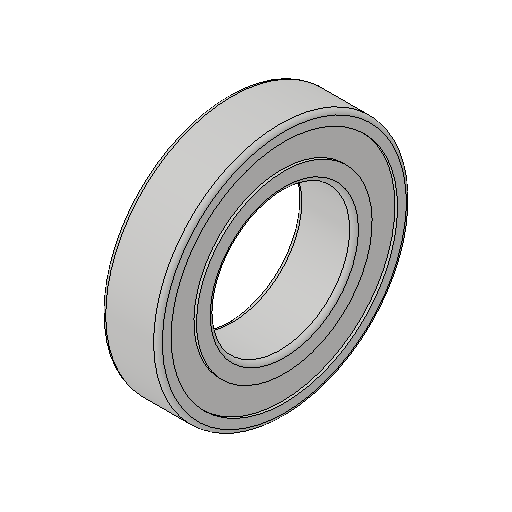
# Autodesk Inventor part: BEARING
Saved by Autodesk Inventor 2022.5 (Build 265521000, 521)
## iProperties
Created: 2023-01-26
Material: 일반
Catalog Web Link: www.cadenas.de
Vendor: MISUMI
Document SubType Name: Modeling
Manufacturer: MISUMI
Mass: 22.7584 g
Surface Area: 74.5546 cm^2
Volume: 22.7584 cm^3
Density: 1 g/cm^3
Appearance: 기본값
Description: 3
Part Number: BEARING
PSOL_IDENT_0: {$CADENAS_DATA/23d-libs/misumi/metric/12_bearing_holders/sb6010zz.prj},174 {VTYP=3D},{NB=B60-32ZZ},{
PSOL_IDENT_1: LINA=B60-32ZZ},{NN=B6_ _ _ZZ, SB6_ _ _ZZ},{DATE=30.06.2021 12:59:24},{GEOMDATE=22.10.2019 06:26:04},
PSOL_IDENT_2: {VERSION=},{LINEID=720},{WBVAR=TS},{WBNUMERIC=}  {NB=B60-32ZZ},{LINA=B60-32ZZ},{KT=DUMMY},{PN=B60-32
PSOL_IDENT_3: ZZ},{TS=},{TS1= '', 'Steel'},{MAT=52100 Bearing Steel},{BN=60-32ZZ},{DD=32},{D=58},{B=13},{RR=1.0},{
PSOL_IDENT_4: CR=11.8},{COR=8.05},{CRS=11.8},{CRSS=-},{CORS=8.05},{CORSS=-},{DD1=0.00},{R1=0.00},{R2=0.0},{DSMIN=3
PSOL_IDENT_5: 7.0},{DSMAX=39.00},{DS1=39.00},{DDHH=53.0},{R=1.0},{MASS=129},{MASS11=129},{AA=11.8040},{BB=3.0044},
PSOL_IDENT_6: {CC=4.1600},{TYS=w/o Retaining Ring}
NB: B60-32ZZ
NN: B6_ _ _ZZ, SB6_ _ _ZZ
NT: Deep Groove Ball Bearings - Double Shield Type
NBSYN: $PN.
LINA: B60-32ZZ
CATALOG: Misumi
PN: B60-32ZZ
TS: Steel
MAT: 52100 Bearing Steel
BN: 60-32ZZ
DD: 32
D: 58
B: 13
RR: 1
CR: 11.8
COR: 8.05
DSMIN: 37
DSMAX: 39
DDHH: 53
R: 1
MASS: 129
SUPPLIER: MISUMI
ARTICLENO: B60-32ZZ
BOMINFO: B60-32ZZ
CREATOR: CADENAS GmbH
MAKER: NSK
Detail Description: Purchased products
Title: 60-32ZZ
Revision Number: A
Autodesk Inventor part; units mm, degrees
sketch "Sketch_1" plane through (0, 0, 0) normal (0, 0, 1) x (1, 0, 0)
  line L0 (13, 0) -> (0, 0)
  arc A0 (0, 17) -> (1, 16) centre (1, 17) ccw
  line L1 (1, 16) -> (12, 16)
  arc A1 (12, 16) -> (13, 17) centre (12, 17) ccw
  line L2 (13, 17) -> (13, 20.16)
  line L3 (13, 20.16) -> (12.402, 20.16)
  line L4 (12.402, 20.16) -> (12.402, 25.9956)
  line L5 (12.402, 25.9956) -> (13, 25.9956)
  line L6 (13, 25.9956) -> (13, 28)
  arc A2 (13, 28) -> (12, 29) centre (12, 28) ccw
  line L7 (12, 29) -> (1, 29)
  arc A3 (1, 29) -> (0, 28) centre (1, 28) ccw
  line L8 (0, 28) -> (0, 25.9956)
  line L9 (0, 25.9956) -> (0.598, 25.9956)
  line L10 (0.598, 25.9956) -> (0.598, 20.16)
  line L11 (0.598, 20.16) -> (0, 20.16)
  line L12 (0, 20.16) -> (0, 17)
  constraints: 26 end point, 8 point on circle, 4 centre point
revolve "Revolution1" add sketch "Sketch_1" angle 360 about axis through (13, 0, 0) along (1, 0, 0)
ref_plane "center_point_XY" through (6.5, 0, 0) normal (1, 0, 0) x (0, 0, -1)
ref_plane "center_point_YZ" through (6.5, 0, 0) normal (0, 0, -1) x (0, 1, 0)
ref_plane "center_point_ZX" through (6.5, 0, 0) normal (0, 1, 0) x (1, 0, 0)
ref_plane "to_housing_XY" through (0, 0, 0) normal (1, 0, 0) x (0, 0, -1)
ref_plane "to_housing_YZ" through (0, 0, 0) normal (0, 0, -1) x (0, 1, 0)
ref_plane "to_housing_ZX" through (0, 0, 0) normal (0, 1, 0) x (1, 0, 0)
ref_plane "to_ring_XY" through (11.804, 0, 0) normal (1, 0, 0) x (0, 0, -1)
ref_plane "to_ring_YZ" through (11.804, 0, 0) normal (0, 0, -1) x (0, 1, 0)
ref_plane "to_ring_ZX" through (11.804, 0, 0) normal (0, 1, 0) x (1, 0, 0)
body "Solid1"
